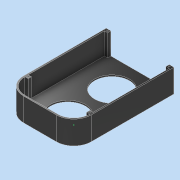
# Autodesk Inventor part: Part1
Saved by Autodesk Inventor 2022 (Build 260153000, 153)
## iProperties
Created: 2022-09-15
Part Number: Part1
Material: Generic
Document SubType Name: Modeling
Designer: aleal
Density: 1 g/cm^3
Appearance: Glossy - Black
Author: aleal
Autodesk Inventor part; units mm, degrees
ref_plane "YZ Plane" through (0, 0, 0) normal (1, 0, 0) x (0, 1, 0)
ref_plane "XZ Plane" through (0, 0, 0) normal (0, 1, 0) x (-1, 0, 0)
ref_plane "XY Plane" through (0, 0, 0) normal (0, 0, 1) x (1, 0, 0)
sketch "Sketch1" plane through (0, 0, 0) normal (0, 1, 0) x (-1, 0, 0)
  line L0 (0, 0) -> (146, 0)
  line L1 (146, 0) -> (146, -216)
  line L2 (146, -216) -> (0, -216)
  line L3 (0, -216) -> (0, 0)
  dimension "d0" = 146
  dimension "d1" = 216
  constraints: 8 end point, 2 parallel, 1 horizontal, 1 perpendicular
  measures "d0" distance of L1.end L2.end
  measures "d1" distance of L0.end L1.end
extrude "Extrusion1" add sketch "Sketch1" along normal blind 50
sketch "Sketch2" plane through (0, 50, 0) normal (0, 1, 0) x (1, 0, 0)
  point P0 (0, 0)
fillet "Fillet1" radius 37.5 2 edges at (-146, 25, 0) (0, 25, 0)
sketch "Sketch3" plane through (0, 50, 0) normal (0, 1, 0) x (1, 0, 0)
  line L0 (0, 216) -> (-146, 216) projected
  line L1 (-146, 216) -> (0, 216)
  line L2 (0, 216) -> (0, 37.5)
  line L3 (-37.5, 0) -> (-108.5, 0)
  line L4 (-146, 37.5) -> (-146, 216)
  arc A0 (-146, 37.5) -> (-108.5, 0) centre (-108.5, 37.5) ccw
  arc A1 (-37.5, 0) -> (0, 37.5) centre (-37.5, 37.5) ccw
  line L5 (-143, 213) -> (-3, 213)
  line L6 (-3, 213) -> (-3, 37.5)
  arc A2 (-37.5, 3) -> (-3, 37.5) centre (-37.5, 37.5) ccw
  line L7 (-37.5, 3) -> (-108.5, 3)
  arc A3 (-143, 37.5) -> (-108.5, 3) centre (-108.5, 37.5) ccw
  line L8 (-143, 37.5) -> (-143, 213)
  point P0 (0, 0)
  dimension "d5" = 37.5
  dimension "d6" = 3
  constraints: 16 end point, 8 point on circle, 4 centre point, 4 parallel, 4 tangent, 2 perpendicular, 2 point on line, 1 equal radius, 1 horizontal, 5 other
  measures "d5" radius of A0
  measures "d6" distance between parallel lines of L4 L8
extrude "Extrusion2" cut sketch "Sketch3" against normal blind 47 contours L5 L6 A2 L7 A3 L8
sketch "Sketch4" plane through (0, 3, 0) normal (0, 1, 0) x (1, 0, 0)
  circle A0 centre (-73, 60.5) radius 37.6
  circle A1 centre (-73, 155.5) radius 37.6
  line L0 (-37.5, 3) -> (-108.5, 3) projected
  line L1 (-3, 213) -> (-3, 37.5) projected
  line L2 (-143, 37.5) -> (-143, 213) projected
  point P0 (0, 0)
  dimension "d9" = 75.2
  dimension "d10" = 75.2
  dimension "d11" = 95
  dimension "d12" = 57.5
  dimension "d13" = 140
  dimension "d14" = 70
  dimension "d15" = 70
  constraints: 2 centre point
  measures "d9" diameter of A0
  measures "d10" diameter of A1
  measures "d11" distance of A1.centre A0.centre
  measures "d12" distance from line of L0 A0.centre
  measures "d13" distance between parallel lines of L1 L2
  measures "d14" distance from line of L2 A0.centre
  measures "d15" distance from line of L2 A1.centre
extrude "Extrusion3" cut sketch "Sketch4" against normal blind 47
sketch "Sketch5" plane through (0, 0, -216) normal (0, 0, -1) x (-1, 0, 0)
  line L0 (3, 50) -> (37.5, 50) projected
  line L1 (108.5, 3) -> (143, 3) projected
  line L2 (3, 50) -> (143, 50)
  line L3 (143, 50) -> (143, 3)
  line L4 (143, 3) -> (3, 3)
  line L5 (3, 3) -> (3, 50)
  point P0 (0, 0)
  point P1 (37.5, 50)
  constraints: 8 end point, 2 parallel, 1 horizontal, 1 perpendicular
extrude "Extrusion4" cut sketch "Sketch5" against normal blind 3
sketch "Sketch6" plane through (0, 50, 0) normal (0, 1, 0) x (1, 0, 0)
  arc A0 (-143, 37.5) -> (-108.5, 3) centre (-108.5, 37.5) ccw projected
  line L0 (-143, 37.5) -> (-136, 37.5)
  line L1 (-136, 37.5) -> (-136, 44.5)
  line L2 (-136, 44.5) -> (-143, 44.5)
  line L3 (-143, 44.5) -> (-143, 37.5)
  line L4 (-3, 37.5) -> (-10, 37.5)
  line L5 (-10, 37.5) -> (-10, 44.5)
  line L6 (-10, 44.5) -> (-3, 44.5)
  line L7 (-3, 44.5) -> (-3, 37.5)
  line L8 (-143, 37.5) -> (-143, 216) projected
  line L9 (-143, 216) -> (-136, 216)
  line L10 (-136, 216) -> (-136, 209)
  line L11 (-136, 209) -> (-143, 209)
  line L12 (-143, 209) -> (-143, 216)
  line L13 (-3, 216) -> (-3, 37.5) projected
  line L14 (-3, 216) -> (-10, 216)
  line L15 (-10, 216) -> (-10, 209)
  line L16 (-10, 209) -> (-3, 209)
  line L17 (-3, 209) -> (-3, 216)
  point P0 (0, 0)
  point P1 (-3, 209)
  dimension "d20" = 7
  dimension "d21" = 7
  dimension "d22" = 7
  dimension "d23" = 7
  dimension "d24" = 7
  dimension "d25" = 7
  dimension "d26" = 7
  dimension "d27" = 7
  constraints: 32 end point, 8 parallel, 4 horizontal, 4 perpendicular
  measures "d20" distance of L2.end L1.end
  measures "d21" distance of L1.end L0.end
  measures "d22" distance of L5.end L6.end
  measures "d23" distance of L4.end L5.end
  measures "d24" distance of L10.end L11.end
  measures "d25" distance of L9.end L10.end
  measures "d26" distance of L16.end L15.end
  measures "d27" distance of L15.end L14.end
extrude "Extrusion5" add sketch "Sketch6" against normal blind 50
sketch "Sketch7" plane through (0, 50, 0) normal (0, 1, 0) x (1, 0, 0)
  circle A0 centre (-139.5, 41) radius 1.45
  line L0 (-136, 44.5) -> (-143, 44.5) projected
  line L1 (-136, 37.5) -> (-136, 44.5) projected
  circle A1 centre (-139.5, 212.5) radius 1.45
  line L2 (-136, 216) -> (-146, 216) projected
  line L3 (-136, 209) -> (-136, 216) projected
  circle A2 centre (-6.5, 212.5) radius 1.45
  line L4 (-10, 216) -> (-10, 209) projected
  line L5 (-10, 209) -> (-3, 209) projected
  circle A3 centre (-6.5, 41) radius 1.45
  line L6 (-10, 44.5) -> (-10, 37.5) projected
  line L7 (-10, 37.5) -> (-3, 37.5) projected
  point P0 (0, 0)
  dimension "d34" = 2.9
  dimension "d35" = 3.5
  dimension "d36" = 3.5
  dimension "d37" = 2.9
  dimension "d38" = 3.5
  dimension "d39" = 3.5
  dimension "d40" = 2.9
  dimension "d41" = 3.5
  dimension "d42" = 3.5
  dimension "d43" = 2.9
  dimension "d44" = 3.5
  dimension "d45" = 3.5
  constraints: 4 centre point
  measures "d34" diameter of A0
  measures "d35" distance from line of L0 A0.centre
  measures "d36" distance from line of L1 A0.centre
  measures "d37" diameter of A1
  measures "d38" distance from line of L2 A1.centre
  measures "d39" distance from line of L3 A1.centre
  measures "d40" diameter of A2
  measures "d41" distance from line of A2.centre L4
  measures "d42" distance from line of L5 A2.centre
  measures "d43" diameter of A3
  measures "d44" distance from line of L6 A3.centre
  measures "d45" distance from line of L7 A3.centre
extrude "Extrusion6" cut sketch "Sketch7" against normal blind 50
equation "\"d14\" = 0.5 * d13"
equation "\"d15\" = d14"
body "Solid1"
